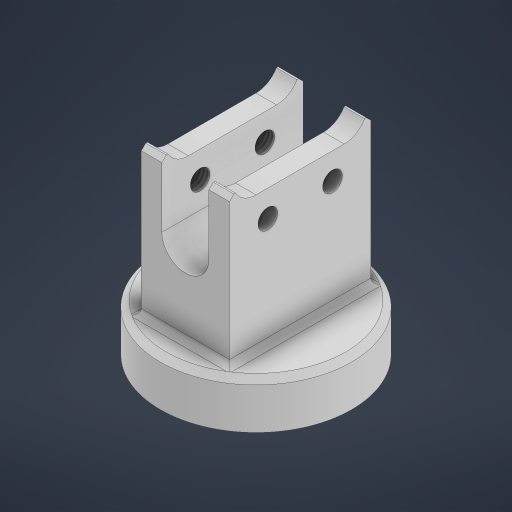
# Autodesk Inventor part: Part5
Saved by Autodesk Inventor 2023.2 (Build 272271000, 271)
## iProperties
Created: 2023-01-17
Part Number: Part5
Material: Generic
Document SubType Name: Modeling
Designer: iusti
Density: 1 g/cm^3
Appearance: Default
Author: iusti
Autodesk Inventor part; units mm, degrees
ref_plane "YZ Plane" through (0, 0, 0) normal (1, 0, 0) x (0, 1, 0)
ref_plane "XZ Plane" through (0, 0, 0) normal (0, 1, 0) x (-1, 0, 0)
ref_plane "XY Plane" through (0, 0, 0) normal (0, 0, 1) x (1, 0, 0)
sketch "Sketch7" plane through (0, 0, 0) normal (0, 0, 1) x (1, 0, 0)
  line L0 (0, 16) -> (32.5, 16)
  line L1 (32.5, 16) -> (32.5, 0)
  line L2 (32.5, 0) -> (27.5, 0)
  line L3 (27.5, 0) -> (27.5, 4)
  line L4 (27.5, 4) -> (22.5, 4)
  line L5 (22.5, 4) -> (22.5, 0)
  line L6 (22.5, 0) -> (18, 0)
  line L7 (18, 0) -> (18, -8)
  line L8 (18, -8) -> (0, -8)
  line L9 (0, 16) -> (0, -8)
  point P0 (0, 0)
  point P1 (22.5, 2)
  dimension "d26" = 16
  dimension "d27" = 32.5
  dimension "d28" = 4
  dimension "d33" = 8
  dimension "d34" = 36
  dimension "d35" = 45
  dimension "d36" = 55
  dimension "d37" = 16
  constraints: 20 end point, 6 perpendicular, 2 horizontal, 1 horizontal alignment, 1 midpoint, 1 point on line, 1 vertical, 1 vertical alignment
  measures "d26" distance of point (0, 0) L0.start
  measures "d27" distance of L0.start L0.end
  measures "d28" distance between parallel lines of L4 L2
  measures "d33" distance of L6.end L7.end
  measures "d34" diameter of L7 L9
  measures "d35" diameter of point (22.5, 2) L9
  measures "d36" diameter of L3 L9
  measures "d37" distance of L0.end L1.end
revolve "Revolution1" add sketch "Sketch7" angle 360 about axis through (0, 16, 0) along (0, -1, 0)
sketch "Sketch10" plane through (0, 0, 0) normal (1, 0, 0) x (0, 1, 0)
  line L0 (16, 32.5) -> (16, -32.5) projected
  line L1 (66, -24) -> (16, -24)
  line L2 (16, -24) -> (16, 24)
  line L3 (16, 24) -> (66, 24)
  line L4 (66, 24) -> (66, 21.9282)
  line L5 (-8, 18) -> (-8, -18) projected
  line L6 (62, -15) -> (62, 15)
  arc A0 (66, 21.9282) -> (62, 15) centre (70, 15) ccw
  line L7 (-23.2262, 0) -> (83.3572, 0) projected
  line L8 (0, 32.5) -> (0, -32.5) projected
  arc A1 (62, -15) -> (66, -21.9282) centre (70, -15) ccw
  line L9 (66, 21.9282) -> (66, -21.9282) construction
  line L10 (66, -21.9282) -> (66, -24)
  point P0 (0, 0)
  point P1 (66, 0)
  point P2 (-8, 0)
  dimension "d49" = 74
  dimension "d52" = 8
  dimension "d53" = 62
  dimension "d54" = 30
  dimension "d56" = 48
  dimension "d57" = 48
  constraints: 14 end point, 4 parallel, 4 point on circle, 3 symmetric about line, 2 centre point, 1 horizontal, 1 horizontal alignment, 1 midpoint, 1 perpendicular, 1 point on line, 1 tangent, 1 vertical, 1 other
  measures "d49" distance between parallel lines of L5 L4
  measures "d52" radius of A0
  measures "d53" distance between parallel lines of L8 L6
  measures "d54" diameter of A0.centre L7
  measures "d56" distance between parallel lines of L1 L3
  measures "d57" diameter of L3 L7
extrude "Extrusion5" add sketch "Sketch10" along normal mid plane 30
sketch "Sketch13" plane through (-15, 16, 24) normal (0, 0, 1) x (1, 0, 0)
  line L0 (0, 50) -> (30, 50) projected
  line L1 (7, 50) -> (7, 28)
  arc A0 (7, 28) -> (23, 28) centre (15, 28) ccw
  line L2 (23, 28) -> (23, 50)
  line L3 (-17.5, -16) -> (47.5, -16) projected
  point P0 (15, -16)
  dimension "d75" = 8
  dimension "d76" = 44
  constraints: 4 end point, 2 perpendicular, 2 point on circle, 2 point on line, 2 tangent, 1 centre point, 1 vertical alignment
  measures "d75" radius of A0
  measures "d76" distance from line of L3 A0.centre
extrude "Extrusion7" cut sketch "Sketch13" against normal through all
chamfer "Chamfer4" distance 1.5 angle 45 4 edges at (-11.5, 66, -24) (11.5, 66, -24) (11.5, 66, 24) (-11.5, 66, 24)
sketch "Sketch14" plane through (0, -8, 0) normal (0, -1, 0) x (1, 0, 0)
  point P0 (0, 0)
hole "Hole1" at (0, -8, 0) direction (0, 1, 0) diameter 22 depth 35 tip angle 118
chamfer "Chamfer5" distance 1.5 angle 45 1 edges at (-18, -8, 0)
chamfer "Chamfer6" distance 2 angle 45 1 edges at (-32.5, 16, 0)
fillet "Fillet2" radius 2 4 edges at (-15, 16, 0) (0, 16, -24) (15, 16, 0) (0, 16, 24)
sketch "Sketch15" plane through (-15, 0, 0) normal (-1, 0, 0) x (0, 0, 1)
  line L0 (-32.5, 0) -> (32.5, 0) projected
  line L1 (0, -23.6) -> (0, 85.6) projected
  point P0 (0, 0)
  point P1 (-11, 53)
  point P2 (11, 53)
  dimension "d97" = 22
  dimension "d98" = 53
  constraints: 1 horizontal alignment, 1 symmetric about line
  measures "d97" distance of point (11, 53) point (-11, 53)
  measures "d98" distance from line of L0 point (11, 53)
hole "Hole2" at (-15, 53, -11) at (-15, 53, 11) direction (1, 0, 0) diameter 6.647 end through all thread size "M8x1.25" class "6H" standard "ISO Metric profile"
body "Solid2"
